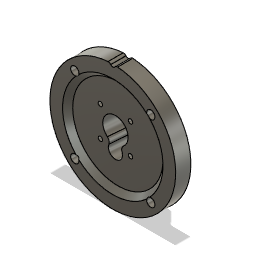
Corsair_Nose v0 (Autodesk Fusion 360 design; units mm, degrees)
Autodesk Fusion 360 part; units mm, degrees
note: some values were not read from the file. Set by a fixed rule: which sketch regions a step uses.
sketch "Skizze1" plane through (0, 0, 0) normal (0, 0, 1) x (1, 0, 0)
  circle A0 centre (0, 0) radius 62
  dimension "d1" = 124
  constraint coincident A0.centre origin
  measures "d1" diameter of A0
extrude "Extrusion1" add sketch "Skizze1" along normal blind 15
sketch "Skizze2" plane through (0, 0, 15) normal (0, 0, 1) x (1, 0, 0)
  circle A0 centre (0, 0) radius 62
  circle A1 centre (0, 0) radius 47
  dimension "d4" = 15
  constraint concentric A0 A1
  measures "d4" distance of A0 A1
extrude "Extrusion2" cut sketch "Skizze2" against normal blind 5 contours A1
chamfer "Fase1" distance 2.5 angle 45 1 edges at (-43.8194, 16.9959, 15)
chamfer "Fase2" distance 2.5 angle 45 1 edges at (-43.8194, 16.9959, 10)
sketch "Skizze3" plane through (0, 0, 0) normal (0, 1, 0) x (1, 0, 0)
  line L0 (0, 0) -> (0, 50) construction
  dimension "d9" = 50
  constraint coincident L0.start origin
  constraint vertical L0
  measures "d9" distance of L0.start L0.end
sketch "Skizze4" plane through (0, 0, 15) normal (0, 0, 1) x (1, 0, 0)
  circle A0 centre (0, 0) radius 62
  circle A1 centre (0, 0) radius 49.5
  circle A2 centre (0, 62) radius 2.5
  dimension "d10" = 5
  constraint vertical A2.centre A0.centre
  constraint coincident A0 A2.centre
  measures "d10" diameter of A2
extrude "Extrusion3" cut sketch "Skizze4" against normal blind 22 contours A0 A2 picked at (-0.0615, 61.1652)
fillet "Abrundung1" radius 3 2 edges at (-2.4995, 61.9496, 7.5) (2.4995, 61.9496, 7.5)
ref_plane "Arbeitsebene1" through (0, -0.0252, -50) normal (0, 0, -1) x (-1, 0, 0)
sketch "Skizze6" plane through (0, 0, 0) normal (0, 1, 0) x (1, 0, 0)
  line L0 (0, 50) -> (-114.5188, 50) construction
  line L1 (-114.5188, 50) -> (0, 45) construction
  line L2 (0, 0) -> (0, 50)
  point P0 (0, 50)
  dimension "d16" = 2.5
  dimension "d17" = 5
  constraint coincident L1.end L2
  constraint coincident P0 L0.start
  constraint horizontal L0
  measures "d16" angle of L0 L1
  measures "d17" distance of L1.end P0
sketch "Skizze7" plane through (0, 0, 0) normal (1, 0, 0) x (0, 0, -1)
  line L0 (50, 0) -> (50, 143.1813) construction
  line L1 (50, 143.1813) -> (45, 0) construction
  point P0 (45, 0)
  point P1 (50, 0)
  dimension "d18" = 2
  constraint coincident P0 L1.end
  constraint coincident L0.start P1
  constraint vertical L0
  measures "d18" angle of L0 L1
sketch "Skizze8" plane through (0, 0, 0) normal (0, 0, -1) x (-1, 0, 0)
  arc A0 (-2.0425, 60.5585) -> (-4.7221, 61.8199) centre (-4.4936, 58.8286) ccw
  arc A1 (-4.7221, 61.8199) -> (4.7221, 61.8199) centre (0, 0) ccw
  arc A2 (4.7221, 61.8199) -> (2.0425, 60.5585) centre (4.4936, 58.8286) ccw
  arc A3 (-2.0425, 60.5585) -> (2.0425, 60.5585) centre (0, 62) ccw
  circle A4 centre (0, 0) radius 40
  dimension "d19" = 80
  constraint coincident A1.centre A4.centre
  measures "d19" diameter of A4
extrude "Extrusion4" add sketch "Skizze8" along normal blind 15 contours A4
ref_plane "Arbeitsebene2" through (-114.5188, 0, -50) normal (0.043593, -0.034866, -0.998441) x (0.624608, 0.780938, 0)
sketch "Skizze9" plane through (-114.5188, 0, -50) normal (0.043593, -0.034866, -0.998441) x (0.624608, 0.780938, 0)
  circle A0 centre (71.5294, 89.5718) radius 26
  point P0 (71.5294, 89.5718)
  dimension "d22" = 52
  constraint coincident P0 A0.centre
  measures "d22" diameter of A0
extrude "Extrusion5" cut sketch "Skizze9" against normal blind 31.5
chamfer "Fase3" distance 12 angle 45 1 edges at (37.2931, -14.4646, -15)
fillet "Abrundung2" radius 5 1 edges at (37.2931, 14.4646, 0)
sketch "Skizze10" plane through (0.5854, -0.4682, -13.4089) normal (0.043593, -0.034866, -0.998441) x (-0.999048, 0, -0.043619)
  circle A0 centre (1.9629, 1.5675) radius 12.5
  line L0 (1.9629, 1.5675) -> (1.9629, 16.0126) construction
  line L1 (16.8121, -13.2818) -> (-12.8864, 16.4167) construction
  line L2 (-12.8864, 16.4167) -> (16.8121, 16.4167) construction
  line L3 (16.8121, 16.4167) -> (-12.8864, -13.2818) construction
  line L4 (-12.8864, 16.4167) -> (-12.8864, -13.2818) construction
  line L5 (16.8121, 16.4167) -> (16.8121, -13.2818) construction
  circle A1 centre (-12.8864, 16.4167) radius 2.15
  circle A2 centre (16.8121, 16.4167) radius 2.15
  circle A3 centre (16.8121, -13.2818) radius 2.15
  circle A4 centre (-12.8864, -13.2818) radius 2.15
  circle A5 centre (1.9629, -16.4325) radius 7
  line L6 (22.6836, 17.2726) -> (21.8626, 18.3007)
  arc A6 (21.8626, 18.3007) -> (22.6836, 17.2726) centre (1.9629, 1.5675) ccw
  dimension "d28" = 25
  dimension "d29" = 42
  dimension "d30" = 4.3
  dimension "d31" = 18
  dimension "d32" = 14
  constraint coincident A0.centre L0.start
  constraint vertical L0
  constraint perpendicular L0 L2
  constraint coincident A0.centre L3
  constraint coincident A0.centre L1
  constraint equal L1 L3
  constraint vertical L4
  constraint vertical L5
  constraint perpendicular L1 L3
  constraint coincident L1.end L2.start
  constraint coincident L2.end L3.start
  constraint coincident L1.start L5.end
  constraint coincident L3.end L4.end
  constraint equal A1 A4
  constraint equal A1 A2
  constraint equal A1 A3
  constraint vertical A0.centre A5.centre
  measures "d28" diameter of A0
  measures "d29" distance of L1.start L1.end
  measures "d30" diameter of A1
  measures "d31" distance of A0.centre A5.centre
  measures "d32" diameter of A5
extrude "Extrusion6" cut sketch "Skizze10" against normal blind 41 contours A0 A5 | A0 A5 | A0 A5 | A1 | A2 | A3 | A4
chamfer "Fase4" distance 5 angle 45 1 edges at (-1.3542, 13.5907, -13.9845)
sketch "Skizze11" plane through (0, 0, 0) normal (0, 0, -1) x (-1, 0, 0)
  arc A0 (-2.0425, 60.5585) -> (-4.7221, 61.8199) centre (-4.4936, 58.8286) ccw
  arc A1 (-4.7221, 61.8199) -> (4.7221, 61.8199) centre (0, 0) ccw
  arc A2 (4.7221, 61.8199) -> (2.0425, 60.5585) centre (4.4936, 58.8286) ccw
  arc A3 (-2.0425, 60.5585) -> (2.0425, 60.5585) centre (0, 62) ccw
  circle A4 centre (0, 0) radius 44.5826
  line L0 (37.5, 37.5) -> (-37.5, 37.5) construction
  line L1 (-37.5, 37.5) -> (-37.5, -37.5) construction
  line L2 (-37.5, -37.5) -> (37.5, -37.5) construction
  line L3 (37.5, -37.5) -> (37.5, 37.5) construction
  line L4 (37.5, 37.5) -> (-37.5, -37.5) construction
  line L5 (-37.5, 37.5) -> (37.5, -37.5) construction
  circle A5 centre (37.5, 37.5) radius 4.1
  circle A6 centre (-37.5, 37.5) radius 4.1
  circle A7 centre (-37.5, -37.5) radius 4.1
  circle A8 centre (37.5, -37.5) radius 4.1
  dimension "d36" = 75
  dimension "d37" = 8.2
  constraint horizontal L0
  constraint perpendicular L0 L1
  constraint parallel L0 L2
  constraint parallel L1 L3
  constraint coincident L4 A1.centre
  constraint coincident L5 A1.centre
  constraint coincident A1.centre A4.centre
  constraint equal L0 L3
  constraint coincident L0.start L3.end
  constraint coincident L0.end L1.start
  constraint coincident L1.end L2.start
  constraint coincident L2.end L3.start
  constraint equal A5 A8
  constraint equal A7 A8
  constraint equal A6 A7
  measures "d36" distance of L0.start L2.end
  measures "d37" diameter of A5
fillet "Abrundung3" radius 5 2 edges at (1.5653, -10.3853, 1.0081) (-5.576, -10.3798, 0.8523)
extrude "Extrusion7" cut sketch "Skizze11" against normal blind 21 contours A5 | A6 | A7 | A8
sketch "Skizze12" plane through (0.5854, -0.4682, -13.4089) normal (0.043593, -0.034866, -0.998441) x (-0.999048, 0, -0.043619)
  line L0 (22.6836, 17.2726) -> (21.8626, 18.3007)
  arc A0 (21.8626, 18.3007) -> (22.6836, 17.2726) centre (1.9629, 1.5675) ccw
  circle A1 centre (-12.8864, 16.4167) radius 2.15
  arc A2 (8.7128, -14.5783) -> (-4.7871, -14.5783) centre (1.9629, 1.5675) ccw
  arc A3 (-4.7871, -14.5783) -> (8.7128, -14.5783) centre (1.9629, -16.4325) ccw
  circle A4 centre (-12.8864, -13.2818) radius 2.15
  circle A5 centre (16.8121, 16.4167) radius 2.15
  circle A6 centre (16.8121, -13.2818) radius 2.15
  line L1 (-37.847, 37.6382) -> (39.4496, 37.6382)
  line L2 (39.4496, 37.6382) -> (39.4496, -38.2551)
  line L3 (39.4496, -38.2551) -> (-37.847, -38.2551)
  line L4 (-37.847, -38.2551) -> (-37.847, 37.6382)
  constraint horizontal L1
  constraint vertical L2
  constraint horizontal L3
  constraint vertical L4
extrude "Extrusion8" cut sketch "Skizze12" along normal blind 20 contours L0 A0 | L1 L2 L3 L4
